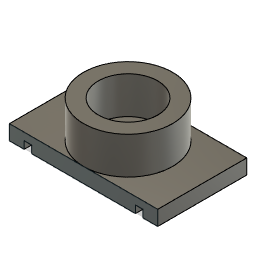
Pen Holder Top v2 (Autodesk Fusion 360 design; units mm, degrees)
Autodesk Fusion 360 part; units mm, degrees
sketch "Sketch1" plane through (0, 0, 0) normal (0, 1, 0) x (1, 0, 0)
  line L0 (0, 0) -> (-20, 0)
  line L1 (-20, 0) -> (-20, 12)
  line L2 (-20, 12) -> (0, 12)
  line L3 (0, 12) -> (0, 0)
  dimension "d1" = 20
  dimension "d2" = 12
  constraint horizontal L0
  constraint vertical L1
  constraint horizontal L2
  constraint vertical L3
  constraint coincident L0.start L3.end
  measures "d1" distance of L0.start L0.end
  measures "d2" distance of L0.start L2.end
extrude "Extrude1" add sketch "Sketch1" along normal blind 2
sketch "Sketch2" plane through (0, 2, 0) normal (0, 1, 0) x (-1, 0, 0)
  line L0 (0, -12) -> (20, -12)
  line L1 (20, -12) -> (20, 0)
  line L2 (20, 0) -> (0, 0)
  line L3 (0, 0) -> (0, -12)
  circle A0 centre (10, -6) radius 5
  circle A1 centre (10, -6) radius 6
  constraint tangent L2 A1
extrude "Extrude2" add sketch "Sketch2" along normal blind 5 contours A1
sketch "Sketch3" plane through (0, 0, 0) normal (0, 0, 1) x (1, 0, 0)
  line L0 (-20, 0) -> (0, 0)
  line L1 (0, 0) -> (0, 2)
  line L2 (0, 2) -> (-10, 2)
  line L3 (-10, 2) -> (-20, 2)
  line L4 (-20, 2) -> (-20, 0)
  line L5 (-17, 0) -> (-18, 0)
  line L6 (-18, 0) -> (-18, 1)
  line L7 (-18, 1) -> (-17, 1)
  line L8 (-17, 1) -> (-17, 0)
  line L9 (-2, 1) -> (-3, 1)
  line L10 (-3, 1) -> (-3, 0)
  line L11 (-3, 0) -> (-2, 0)
  line L12 (-2, 0) -> (-2, 1)
  constraint horizontal L5
  constraint vertical L6
  constraint horizontal L7
  constraint vertical L8
  constraint coincident L0 L5.start
  constraint horizontal L9
  constraint vertical L10
  constraint horizontal L11
  constraint vertical L12
  constraint coincident L0 L10.end
extrude "Extrude3" cut sketch "Sketch3" against normal blind 13 contours L0 L5 L6 L7 L8 | L0 L9 L10 L11 L12
sketch "Sketch4" plane through (0, 0, 0) normal (0, 0, 1) x (1, 0, 0)
  line L0 (-17, 1) -> (-17, 0)
  line L1 (-17, 0) -> (-3, 0)
  line L2 (-3, 0) -> (-3, 1)
  line L3 (-3, 1) -> (-2, 1)
  line L4 (-2, 1) -> (-2, 0)
  line L5 (-2, 0) -> (0, 0)
  line L6 (0, 0) -> (0, 2)
  line L7 (0, 2) -> (-10, 2)
  line L8 (-10, 2) -> (-20, 2)
  line L9 (-20, 2) -> (-20, 0)
  line L10 (-20, 0) -> (-18, 0)
  line L11 (-18, 0) -> (-18, 1)
  line L12 (-18, 1) -> (-17, 1)
sketch "Sketch5" plane through (0, 2, 0) normal (0, 1, 0) x (-1, 0, 0)
  circle A0 centre (10, -6) radius 5
  circle A1 centre (10, -6) radius 5
  circle A2 centre (10, -6) radius 4
  constraint tangent A0 A1
extrude "Extrude4" add sketch "Sketch5" along normal blind 5
